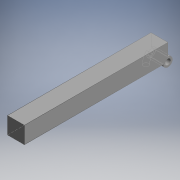
# Autodesk Inventor part: Key0
Saved by Autodesk Inventor 2018 (Build 220112000, 112)
## iProperties
Created: 2018-10-01
Part Number: Key0
Material: Generic
Document SubType Name: Modeling
Designer: Isaac Newcomb
Density: 1 g/cm^3
Appearance: Default
SweepAngle: 42.97 deg
SweepRadius: 8.000 mm
RingThickness: 3.000 mm
Author: Isaac Newcomb
Autodesk Inventor part; units mm, degrees
ref_plane "YZ Plane" through (0, 0, 0) normal (1, 0, 0) x (0, 1, 0)
ref_plane "XZ Plane" through (0, 0, 0) normal (0, 1, 0) x (-1, 0, 0)
sketch "Base" plane through (0, 0, 0) normal (0, 1, 0) x (-1, 0, 0)
  line L0 (0, 0) -> (-10, 0)
  line L1 (-10, 0) -> (-10, 85)
  line L2 (-10, 85) -> (0, 85)
  line L3 (0, 85) -> (0, 0)
  dimension "KeyWidth" = 10
  dimension "KeyLength" = 85
  constraints: 8 end point, 2 parallel, 1 horizontal, 1 perpendicular
  measures "KeyWidth" distance of L1.end L2.end
  measures "KeyLength" distance of L0.end L1.end
extrude "Main Body" add sketch "Base" along normal blind 10
sketch "Hinge Sketch" plane through (10, 0, 85) normal (1, 0, 0) x (0, 0, -1)
  circle A0 centre (85, 0) radius 1.7
  circle A1 centre (85, 0) radius 2.7
  dimension "d10" = 3.4
  dimension "d11" = 1
  constraints: 2 centre point, 2 coincident
  measures "d10" diameter of A0
  measures "d11" radial gap between concentric circles of A0 A1
extrude "Hinge Surround" add sketch "Hinge Sketch" against normal up to surface (10 mm away)
extrude "Hinge Hole" cut sketch "Hinge Sketch" against normal up to next contours A0
ref_plane "Work Plane1" through (5, 0, 85) normal (1, 0, 0) x (0, 0, -1)
sketch "Sweep Path" plane through (5, 0, 85) normal (1, 0, 0) x (0, 0, -1)
  arc A0 (79.1465, 5.4531) -> (77, 0) centre (85, 0) ccw
  line L0 (0, 0) -> (82.3, 0) construction
  dimension "SweepAngle" = 42.972
  dimension "SweepRadius" = 8
  constraints: 2 point on circle, 1 centre point, 1 coincident, 1 point on line
  measures "SweepRadius" radius of A0
sketch "Sweep Profile" plane through (0, 0, 0) normal (0, -1, 0) x (1, 0, 0)
  circle A0 centre (5, 8) radius 1.5
  point P0 (0, 0)
  dimension "RingThickness" = 3
  constraints: 1 centre point, 1 coincident
  measures "RingThickness" diameter of A0
sweep "Sweep2" cut profiles "Sweep Profile" path "Sweep Path"
equation "\"KeyWidth\" = MaxWidth"
equation "\"SweepArcLength\" = 6"
equation "\"MaxWidth\" = 10"
body "Solid1"
